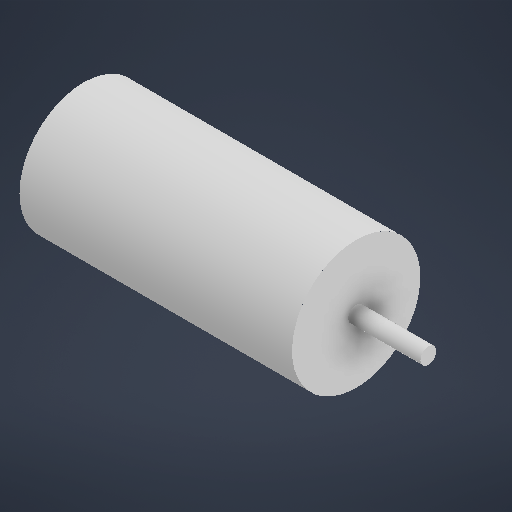
# Autodesk Inventor part: Мотор 17x8
Saved by Autodesk Inventor 2026.2 (Build 302298000, 298)
## iProperties
Created: 2026-02-21
Part Number: Мотор 17x8
Material: Типовые
Document SubType Name: Modeling
Designer: Leonid
Density: 1 g/cm^3
Appearance: По умолчанию
Author: Leonid
Autodesk Inventor part; units mm, degrees
ref_plane "YZ Plane" through (0, 0, 0) normal (1, 0, 0) x (0, 1, 0)
ref_plane "XZ Plane" through (0, 0, 0) normal (0, 1, 0) x (-1, 0, 0)
ref_plane "XY Plane" through (0, 0, 0) normal (0, 0, 1) x (1, 0, 0)
sketch "Эскиз1" plane through (0, 0, 0) normal (1, 0, 0) x (0, 1, 0)
  circle A0 centre (0, 0) radius 4
  circle A1 centre (0, 0) radius 0.5
  dimension "d0" = 8
  dimension "d1" = 1
  constraints: 2 centre point, 2 coincident
  measures "d0" diameter of A0
  measures "d1" diameter of A1
extrude "Выдавливание1" add sketch "Эскиз1" against normal blind 17 contours A0 | A1
extrude "Выдавливание2" add sketch "Эскиз1" along normal blind 4.5 contours A1
